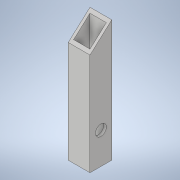
# Autodesk Inventor part: BottomStorageSupport.ver1-1111-2020
Saved by Autodesk Inventor 2021 (Build 250183000, 183)
## iProperties
Created: 2020-01-20
Part Number: BottomStorageSupport.ver1-1111-2020
Material: Generic
Document SubType Name: Modeling
Designer: JMHal
Density: 1 g/cm^3
Appearance: Default
Author: JMHal
Autodesk Inventor part; units mm, degrees
ref_plane "YZ Plane" through (0, 0, 0) normal (1, 0, 0) x (0, 1, 0)
ref_plane "XZ Plane" through (0, 0, 0) normal (0, 1, 0) x (-1, 0, 0)
ref_plane "XY Plane" through (0, 0, 0) normal (0, 0, 1) x (1, 0, 0)
sketch "Sketch1" plane through (0, 0, 0) normal (0, 1, 0) x (-1, 0, 0)
  line L0 (0, 0) -> (25.4, 0)
  line L1 (25.4, 0) -> (25.4, -25.4)
  line L2 (25.4, -25.4) -> (0, -25.4)
  line L3 (0, -25.4) -> (0, 0)
  line L4 (22.225, -22.225) -> (22.225, -3.175)
  line L5 (22.225, -3.175) -> (3.175, -3.175)
  line L6 (3.175, -3.175) -> (3.175, -22.225)
  line L7 (3.175, -22.225) -> (22.225, -22.225)
  dimension "d0" = 25.4
  dimension "d1" = 25.4
  dimension "d2" = 3.175
  constraints: 16 end point, 4 parallel, 2 perpendicular, 1 horizontal, 3 other
  measures "d0" distance of L1.end L2.end
  measures "d1" distance of L0.end L1.end
  measures "d2" distance between parallel lines of L1 L4
extrude "Extrusion1" add sketch "Sketch1" along normal blind 141.7828
sketch "Sketch2" plane through (0, 0, 0) normal (1, 0, 0) x (0, 0, -1)
  line L0 (25.4, 0) -> (0, 0) projected
  line L1 (25.4, 0) -> (25.4, 141.7828) projected
  line L2 (0, 141.7828) -> (25.4, 141.7828) projected
  line L3 (0, 0) -> (0, 141.7828) projected
  line L4 (0, 141.7828) -> (25.4, 141.7828)
  line L5 (25.4, 141.7828) -> (25.4, 118.9125)
  line L6 (25.4, 118.9125) -> (0, 118.9125)
  line L7 (0, 118.9125) -> (0, 141.7828)
  line L8 (25.4, 0) -> (25.4, 141.7828) projected
  line L9 (25.4, 141.7828) -> (0, 118.9125)
  dimension "d5" = 48
  constraints: 10 end point, 2 parallel, 1 horizontal, 1 perpendicular, 1 point on line
  measures "d5" angle of L3 L9
extrude "Extrusion2" cut sketch "Sketch2" against normal blind 141.7828 contours L3 L2 L9
sketch "Sketch3" plane through (0, 0, 0) normal (1, 0, 0) x (0, 0, -1)
  line L0 (25.4, 0) -> (25.4, 73.406)
  circle A0 centre (12.7, 36.703) radius 6.35
  line L1 (25.4, 0) -> (0, 0) projected
  dimension "d8" = 73.406
  dimension "d10" = 12.7
  dimension "d12" = 36.703
  constraints: 2 end point, 1 centre point
  measures "d8" distance of L0.start L0.end
  measures "d10" diameter of A0
  measures "d12" distance from line of L1 A0.centre
extrude "Extrusion3" cut sketch "Sketch3" against normal blind 25.4
body "Solid1"
